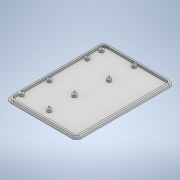
# Autodesk Inventor part: Base
Saved by Autodesk Inventor 2022 (Build 260153000, 153)
## iProperties
Created: 2021-07-02
Part Number: Base
Material: Generic
Document SubType Name: Modeling
Designer: anton
Density: 1 g/cm^3
Appearance: Default
Author: anton
Autodesk Inventor part; units mm, degrees
ref_plane "YZ Plane" through (0, 0, 0) normal (1, 0, 0) x (0, 1, 0)
ref_plane "XZ Plane" through (0, 0, 0) normal (0, 1, 0) x (-1, 0, 0)
ref_plane "XY Plane" through (0, 0, 0) normal (0, 0, 1) x (1, 0, 0)
sketch "Sketch1" plane through (0, 0, 0) normal (0, 1, 0) x (-1, 0, 0)
  line L0 (8.7167, -6) -> (127.3869, -6)
  ellipse E0 centre (8.7167, 0) end of major axis (15.2542, 0) minor radius 6 (2.1792, 0) -> (8.7167, -6) ccw
  line L1 (2.1792, 177.2) -> (2.1792, 0)
  ellipse E1 centre (8.7167, 177.2) end of major axis (15.2542, 177.2) minor radius 6 (8.7167, 183.2) -> (2.1792, 177.2) ccw
  line L2 (127.3869, 183.2) -> (8.7167, 183.2)
  ellipse E2 centre (127.3869, 175.2) end of major axis (137.4774, 175.2) minor radius 8 (137.4774, 175.2) -> (127.3869, 183.2) ccw
  line L3 (137.4774, 175.2) -> (137.4774, 2)
  ellipse E3 centre (127.3869, 2) end of major axis (117.2964, 2) minor radius 8 (127.3869, -6) -> (137.4774, 2) ccw
  ellipse E4 centre (129.9095, 0) end of major axis (140, 0) minor radius 8 (129.9095, -8) -> (140, 0) ccw
  line L4 (140, 177.2) -> (140, 0)
  ellipse E5 centre (129.9095, 177.2) end of major axis (140, 177.2) minor radius 8 (140, 177.2) -> (129.9095, 185.2) ccw
  line L5 (8.7167, 185.2) -> (129.9095, 185.2)
  ellipse E6 centre (8.7167, 177.2) end of major axis (0, 177.2) minor radius 8 (8.7167, 185.2) -> (0, 177.2) ccw
  line L6 (0, 0) -> (0, 177.2)
  ellipse E7 centre (8.7167, 0) end of major axis (0, 0) minor radius 8 (0, 0) -> (8.7167, -8) ccw
  line L7 (129.9095, -8) -> (8.7167, -8)
  line L8 (127.3869, 180.2) -> (8.7167, 180.2)
  line L9 (5.1792, 177.2) -> (5.1792, 0)
  line L10 (8.7167, -3) -> (127.3869, -3)
  line L11 (134.4774, 2) -> (134.4774, 175.2)
  spline S0 degree 5 poles (8.7167, 180.2) (8.1502, 180.1999) (7.5837, 180.1027) (7.0396, 179.9088) (6.1327, 179.3761) (5.4975, 178.5497) (5.2854, 178.1225) (5.1792, 177.6615) (5.1792, 177.2) knots 0 0 0 0 0 0 0.551144 0.551144 0.551144 1 1 1 1 1 1
  spline S1 degree 5 poles (5.1792, 0) (5.1792, -0.4615) (5.2854, -0.9225) (5.4975, -1.3497) (6.1327, -2.1761) (7.0396, -2.7088) (7.5837, -2.9027) (8.1502, -2.9999) (8.7167, -3) knots 0 0 0 0 0 0 0.448856 0.448856 0.448856 1 1 1 1 1 1
  spline S2 degree 5 poles (127.3869, -3) (128.0574, -3) (128.728, -2.9422) (129.3919, -2.8265) (130.8557, -2.4338) (132.2004, -1.7239) (132.8895, -1.2301) (133.7795, -0.3215) (134.2977, 0.8116) (134.4173, 1.1998) (134.4774, 1.5998) (134.4774, 2) knots 0 0 0 0 0 0 0.351315 0.351315 0.351315 0.790279 0.790279 0.790279 1 1 1 1 1 1
  spline S3 degree 5 poles (134.4774, 175.2) (134.4774, 175.6002) (134.4173, 176.0002) (134.2977, 176.3884) (133.7795, 177.5215) (132.8895, 178.4301) (132.2004, 178.9239) (130.8557, 179.6338) (129.3919, 180.0265) (128.728, 180.1422) (128.0574, 180.2) (127.3869, 180.2) knots 0 0 0 0 0 0 0.209721 0.209721 0.209721 0.648685 0.648685 0.648685 1 1 1 1 1 1
  point P0 (96.2591, -8)
  dimension "d3" = 3
  constraints: 24 end point, 7 parallel, 44 other
extrude "Extrusion1" add sketch "Sketch1" along normal blind 6 contours E0 L1 E1 L2 E2 L3 E3 L0
sketch "Sketch4" plane through (0, 0, 0) normal (0, 1, 0) x (-1, 0, 0)
  ellipse E0 centre (129.9095, 0) end of major axis (140, 0) minor radius 8 (129.9095, -8) -> (140, 0) ccw
  line L0 (140, 177.2) -> (140, 0)
  ellipse E1 centre (129.9095, 177.2) end of major axis (140, 177.2) minor radius 8 (140, 177.2) -> (129.9095, 185.2) ccw
  line L1 (8.7167, 185.2) -> (129.9095, 185.2)
  ellipse E2 centre (8.7167, 177.2) end of major axis (0, 177.2) minor radius 8 (8.7167, 185.2) -> (0, 177.2) ccw
  line L2 (0, 0) -> (0, 177.2)
  ellipse E3 centre (8.7167, 0) end of major axis (0, 0) minor radius 8 (0, 0) -> (8.7167, -8) ccw
  line L3 (129.9095, -8) -> (8.7167, -8)
  point P0 (96.2591, -8)
  constraints: 8 end point, 16 other
extrude "Extrusion2" add sketch "Sketch4" along normal blind 2
sketch "Sketch5" plane through (0, 2, 0) normal (0, 1, 0) x (1, 0, 0)
  line L0 (-68.42, -103.05) -> (-140, -103.05)
  line L1 (-140, -103.05) -> (-140, -170.2)
  line L2 (-140, -170.2) -> (-68.42, -170.2)
  line L3 (-68.42, -170.2) -> (-68.42, -103.05)
  circle A0 centre (-77.953, -111.49) radius 4
  circle A1 centre (-77.104, -162.39) radius 4
  circle A2 centre (-128.105, -110.86) radius 4
  circle A3 centre (-131.398, -162.39) radius 4
  line L4 (-140, 0) -> (-140, -177.2) projected
  line L5 (-8.7167, 8) -> (-129.9095, 8) projected
  line L6 (-8.7167, -180.2) -> (-127.3869, -180.2) projected
  point P0 (0, 0)
  dimension "d12" = 71.58
  dimension "d13" = 67.15
  dimension "d14" = 8
  dimension "d15" = 8
  dimension "d16" = 8
  dimension "d17" = 8
  dimension "d18" = 8.44
  dimension "d19" = 7.81
  dimension "d20" = 9.533
  dimension "d21" = 8.684
  dimension "d22" = 11.895
  dimension "d23" = 7.81
  dimension "d24" = 7.81
  dimension "d25" = 8.602
  dimension "d26" = 0
  dimension "d28" = 10
  constraints: 8 end point, 4 centre point, 2 parallel, 1 horizontal, 1 perpendicular
  measures "d12" distance between parallel lines of L1 L3
  measures "d13" distance between parallel lines of L2 L0
  measures "d14" diameter of A0
  measures "d15" diameter of A1
  measures "d16" diameter of A3
  measures "d17" diameter of A2
  measures "d18" distance from line of L0 A0.centre
  measures "d19" distance from line of L2 A1.centre
  measures "d20" distance from line of L3 A0.centre
  measures "d21" distance from line of L3 A1.centre
  measures "d22" distance from line of L1 A2.centre
  measures "d23" distance from line of L0 A2.centre
  measures "d24" distance from line of L2 A3.centre
  measures "d25" distance from line of L1 A3.centre
  measures "d26" distance between parallel lines of L4 L1
  measures "d28" distance between parallel lines of L6 L2
extrude "Extrusion3" add sketch "Sketch5" along normal blind 4 contours A0 | A1 | A2 | A3
sketch "Sketch6" plane through (-77.953, 6, 111.49) normal (0, 1, 0) x (1, 0, 0)
  circle A0 centre (0, 0) radius 4 projected
  circle A1 centre (0, 0) radius 1.25
  circle A2 centre (-50.152, 0.63) radius 4 projected
  circle A3 centre (-50.152, 0.63) radius 1.25
  arc A4 (-56.5244, -53.4529) -> (-56.5244, -48.3471) centre (-53.445, -50.9) ccw projected
  circle A5 centre (-53.445, -50.9) radius 1.25
  circle A6 centre (0.849, -50.9) radius 4 projected
  circle A7 centre (0.849, -50.9) radius 1.25
  point P0 (77.953, 111.49)
  dimension "d31" = 2.5
  dimension "d32" = 2.5
  dimension "d33" = 2.5
  dimension "d34" = 2.5
  constraints: 4 centre point, 4 coincident
  measures "d31" diameter of A5
  measures "d32" diameter of A7
  measures "d33" diameter of A1
  measures "d34" diameter of A3
extrude "Extrusion4" add sketch "Sketch6" along normal blind 4 contours A1 | A3 | A5 | A7
sketch "Sketch7" plane through (0, 2, 0) normal (0, 1, 0) x (1, 0, 0)
  line L0 (-130.1792, -53) -> (-55.1792, -53)
  line L1 (-55.1792, -53) -> (-55.1792, 0)
  line L2 (-55.1792, 0) -> (-130.1792, 0)
  line L3 (-130.1792, 0) -> (-130.1792, -53)
  circle A0 centre (-128.1792, -35.7) radius 4
  circle A1 centre (-128.1792, -7.6) radius 4
  circle A2 centre (-69.8792, -50.9) radius 4
  circle A3 centre (-68.8792, -2.1) radius 4
  line L4 (-140, 0) -> (-140, -177.2) projected
  line L5 (-8.7167, 8) -> (-129.9095, 8) projected
  line L6 (-134.4774, -159.8371) -> (-134.4774, -2) projected
  line L7 (-5.1792, 0) -> (-5.1792, -177.2) projected
  point P0 (0, 0)
  dimension "d37" = 75
  dimension "d38" = 53
  dimension "d39" = 8
  dimension "d40" = 8
  dimension "d41" = 8
  dimension "d42" = 8
  dimension "d43" = 14.7
  dimension "d44" = 2.1
  dimension "d45" = 2.1
  dimension "d46" = 13.7
  dimension "d47" = 2
  dimension "d48" = 2
  dimension "d49" = 7.6
  dimension "d50" = 17.3
  dimension "d53" = 8
  dimension "d55" = 50
  constraints: 8 end point, 4 centre point, 2 parallel, 1 perpendicular
  measures "d37" distance between parallel lines of L1 L3
  measures "d38" distance between parallel lines of L2 L0
  measures "d39" diameter of A0
  measures "d40" diameter of A1
  measures "d41" diameter of A3
  measures "d42" diameter of A2
  measures "d43" distance from line of L1 A2.centre
  measures "d44" distance from line of L0 A2.centre
  measures "d45" distance from line of L2 A3.centre
  measures "d46" distance from line of L1 A3.centre
  measures "d47" distance from line of L3 A0.centre
  measures "d48" distance from line of L3 A1.centre
  measures "d49" distance from line of L2 A1.centre
  measures "d50" distance from line of L0 A0.centre
  measures "d53" distance between parallel lines of L5 L2
  measures "d55" distance between parallel lines of L7 L1
extrude "Extrusion5" add sketch "Sketch7" along normal blind 4 contours A2 L0 | L0 A2 | A0 L3 | L3 A0 | A1 L3 | L3 A1 | A3 L2 | L2 A3
sketch "Sketch8" plane through (-68.8792, 6, 2.1) normal (0, 1, 0) x (1, 0, 0)
  circle A0 centre (0, 0) radius 1.25
  circle A1 centre (-1, -48.8) radius 4 projected
  circle A2 centre (-1, -48.8) radius 1.25
  circle A3 centre (-59.3, -33.6) radius 4 projected
  circle A4 centre (-59.3, -33.6) radius 1.25
  circle A5 centre (-59.3, -5.5) radius 4 projected
  circle A6 centre (-59.3, -5.5) radius 1.25
  point P0 (68.8792, 2.1)
  dimension "d58" = 2.5
  dimension "d59" = 2.5
  dimension "d60" = 2.5
  dimension "d61" = 2.5
  constraints: 4 centre point, 3 coincident
  measures "d58" diameter of A6
  measures "d59" diameter of A4
  measures "d60" diameter of A2
  measures "d61" diameter of A0
extrude "Extrusion6" add sketch "Sketch8" along normal blind 4 contours A0 | A2 | A4 | A6
body "Solid1"
